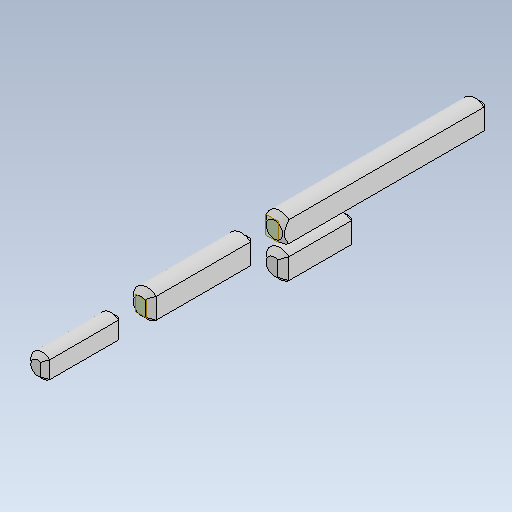
# Autodesk Inventor part: pins
Saved by Autodesk Inventor 2023 (Build 270158030, 158C)
## iProperties
Created: 2024-12-20
Part Number: pins
Material: Generic
Document SubType Name: Modeling
Designer: Imogen Heard
Density: 1 g/cm^3
Appearance: Default
Author: Imogen Heard
Autodesk Inventor part; units mm, degrees
ref_plane "YZ Plane" through (0, 0, 0) normal (1, 0, 0) x (0, 1, 0)
ref_plane "XZ Plane" through (0, 0, 0) normal (0, 1, 0) x (-1, 0, 0)
ref_plane "XY Plane" through (0, 0, 0) normal (0, 0, 1) x (1, 0, 0)
sketch "Sketch1" plane through (0, 0, 0) normal (0, 0, 1) x (1, 0, 0)
  circle A0 centre (-1.65, -26) radius 2.5
  line L0 (-1.65, -28.5) -> (0, -28.5)
  line L1 (0, -28.5) -> (0, -23.5)
  line L2 (0, -23.5) -> (-1.65, -23.5)
  line L3 (-1.65, -23.5) -> (-1.65, -28.5)
  circle A1 centre (-1.65, -38) radius 2.5
  line L4 (-1.65, -40.5) -> (0, -40.5)
  line L5 (0, -40.5) -> (0, -35.5)
  line L6 (0, -35.5) -> (-1.65, -35.5)
  line L7 (-1.65, -35.5) -> (-1.65, -40.5)
  circle A2 centre (-1.65, -44) radius 2.5
  line L8 (-1.65, -46.5) -> (0, -46.5)
  line L9 (0, -46.5) -> (0, -41.5)
  line L10 (0, -41.5) -> (-1.65, -41.5)
  line L11 (-1.65, -41.5) -> (-1.65, -46.5)
  circle A3 centre (-1.65, -32) radius 2.5
  line L12 (-1.65, -34.5) -> (0, -34.5)
  line L13 (0, -34.5) -> (0, -29.5)
  line L14 (0, -29.5) -> (-1.65, -29.5)
  line L15 (-1.65, -29.5) -> (-1.65, -34.5)
  point P0 (0, 0)
  point P1 (0, -27.8782)
  point P2 (0, -24.1218)
  point P3 (0, -33.8782)
  point P4 (0, -30.1218)
  point P5 (0, -39.8782)
  point P6 (0, -36.1218)
  point P7 (0, -45.8782)
  point P8 (0, -42.1218)
  dimension "d0" = 5
  dimension "d1" = 26
  dimension "d2" = 1.65
  dimension "d3" = 5
  dimension "d4" = 1.65
  dimension "d5" = 5
  dimension "d6" = 1.65
  dimension "d7" = 5
  dimension "d8" = 1.65
  dimension "d9" = 6
  dimension "d10" = 6
  dimension "d11" = 6
  constraints: 32 end point, 8 parallel, 8 point on circle, 8 vertical alignment, 4 centre point, 4 horizontal, 4 midpoint, 4 perpendicular
  measures "d0" diameter of A0
  measures "d1" vertical distance of point (0, 0) point (-1.65, -26)
  measures "d2" distance between parallel lines of L1 L3
  measures "d3" diameter of A1
  measures "d4" distance between parallel lines of L5 L7
  measures "d5" diameter of A2
  measures "d6" distance between parallel lines of L9 L11
  measures "d7" diameter of A3
  measures "d8" distance between parallel lines of L13 L15
  measures "d9" distance of A3.centre A0.centre
  measures "d10" distance of point (-1.65, -38) A3.centre
  measures "d11" distance of A1.centre A2.centre
extrude "Extrusion1" add sketch "Sketch1" against normal blind 17 contours L3 A0 | A0 L1 L3
chamfer "Chamfer1" distance 1 angle 45 4 edges at (0, -26, 0) (-4.15, -26, 0) (0, -26, -17) (-4.15, -26, -17)
ref_plane "Work Plane1" through (0, 0, -23) normal (0, 0, -1) x (-1, 0, 0)
sketch "Sketch2" plane through (0, 0, -23) normal (0, 0, -1) x (-1, 0, 0)
  circle A0 centre (1.98, -26) radius 3
  line L0 (1.98, -23) -> (0, -23)
  line L1 (0, -23) -> (0, -29)
  line L2 (0, -29) -> (1.98, -29)
  line L3 (1.98, -29) -> (1.98, -23)
  line L4 (1, -27.3519) -> (1, -24.6481) projected
  circle A1 centre (1.98, -33) radius 3
  line L5 (1.98, -30) -> (0, -30)
  line L6 (0, -30) -> (0, -36)
  line L7 (0, -36) -> (1.98, -36)
  line L8 (1.98, -36) -> (1.98, -30)
  line L9 (1.98, -30) -> (1.98, -36)
  circle A2 centre (1.98, -40) radius 3
  line L10 (1.98, -37) -> (0, -37)
  line L11 (0, -37) -> (0, -43)
  line L12 (0, -43) -> (1.98, -43)
  line L13 (1.98, -43) -> (1.98, -37)
  circle A3 centre (1.98, -47) radius 3
  line L14 (1.98, -44) -> (0, -44)
  line L15 (0, -44) -> (0, -50)
  line L16 (0, -50) -> (1.98, -50)
  line L17 (1.98, -50) -> (1.98, -44)
  line L18 (1.98, -44) -> (1.98, -50)
  line L19 (0, -24.1218) -> (0, -27.8782) projected
  point P0 (0, 0)
  point P1 (1, -26)
  point P2 (0, -26.8782)
  point P3 (1.98, -26)
  point P4 (0, -26.8782)
  point P5 (2.0578, -40)
  point P6 (0, -25.8782)
  point P7 (0, -44.7462)
  point P8 (0, -49.2538)
  point P9 (0, -37.7462)
  point P10 (0, -42.2538)
  point P11 (0, -30.7462)
  point P12 (0, -35.2538)
  point P13 (0, -23.7462)
  point P14 (0, -28.2538)
  dimension "d18" = 6
  dimension "d19" = 1.98
  dimension "d20" = 6
  dimension "d21" = 1.98
  dimension "d22" = 7
  dimension "d23" = 6
  dimension "d24" = 1.98
  dimension "d25" = 6
  dimension "d26" = 1.98
  dimension "d27" = 7
  dimension "d28" = 7
  constraints: 36 end point, 11 vertical alignment, 8 parallel, 8 point on circle, 7 midpoint, 6 coincident, 4 centre point, 4 horizontal, 4 perpendicular, 2 horizontal alignment, 2 vertical
  measures "d18" diameter of A0
  measures "d19" distance between parallel lines of L1 L3
  measures "d20" diameter of A1
  measures "d21" distance between parallel lines of L6 L8
  measures "d22" distance of point (1.98, -33) point (1.98, -26)
  measures "d23" diameter of A2
  measures "d24" distance between parallel lines of L11 L13
  measures "d25" diameter of A3
  measures "d26" distance between parallel lines of L15 L17
  measures "d27" distance of point (1.98, -47) point (1.98, -40)
  measures "d28" vertical distance of point (2.058, -40) A1.centre
extrude "Extrusion2" add sketch "Sketch2" along normal blind 23 separate body contours A0 L3 | L3 A0 L1
chamfer "Chamfer2" distance 1.2 angle 45 4 edges at (-4.98, -26, -23) (0, -26, -23) (-4.98, -26, -46) (0, -26, -46)
ref_plane "Work Plane2" through (0, 0, -52) normal (0, 0, -1) x (-1, 0, 0)
sketch "Sketch3" plane through (0, 0, -52) normal (0, 0, -1) x (-1, 0, 0)
  arc A0 (0, -28.2538) -> (0, -23.7462) centre (1.98, -26) ccw projected
  arc A1 (1.2, -27.6222) -> (1.2, -24.3778) centre (1.98, -26) ccw projected
  line L0 (0, -23.7462) -> (0, -28.2538) projected
  line L1 (1.2, -27.6222) -> (1.2, -24.3778) projected
  arc A2 (0, -35.2538) -> (0, -30.7462) centre (1.98, -33) ccw projected
  arc A3 (1.2, -34.6222) -> (1.2, -31.3778) centre (1.98, -33) ccw projected
  line L2 (1.2, -34.6222) -> (1.2, -31.3778) projected
  arc A4 (1.2, -34.6222) -> (1.2, -31.3778) centre (1.98, -33) ccw projected
  line L3 (1.2, -34.6222) -> (1.2, -31.3778) projected
  line L4 (0, -30.7462) -> (0, -35.2538) projected
  point P0 (0, 0)
  constraints: 6 other
extrude "Extrusion3" add sketch "Sketch3" along normal blind 45 separate body contours L0 A0 | L1 A1
sketch "Sketch4" plane through (0, 0, -52) normal (0, 0, 1) x (1, 0, 0)
  line L0 (0, -35.2538) -> (0, -30.7462) projected
  line L1 (-1.2, -34.6222) -> (-1.2, -31.3778) projected
  arc A0 (-1.2, -31.3778) -> (-1.2, -34.6222) centre (-1.98, -33) ccw projected
  arc A1 (0, -30.7462) -> (0, -35.2538) centre (-1.98, -33) ccw projected
  arc A2 (-1.2, -31.3778) -> (-1.2, -34.6222) centre (-1.98, -33) ccw projected
  line L2 (-1.2, -34.6222) -> (-1.2, -31.3778) projected
  line L3 (0, -30.7462) -> (0, -35.2538) projected
  arc A3 (0, -37.7462) -> (0, -42.2538) centre (-1.98, -40) ccw projected
  arc A4 (-1.2, -38.3778) -> (-1.2, -41.6222) centre (-1.98, -40) ccw projected
  line L4 (-1.2, -41.6222) -> (-1.2, -38.3778) projected
  arc A5 (-1.2, -38.3778) -> (-1.2, -41.6222) centre (-1.98, -40) ccw projected
  line L5 (-1.2, -41.6222) -> (-1.2, -38.3778) projected
  line L6 (0, -37.7462) -> (0, -42.2538) projected
  point P0 (0, 0)
  point P1 (0, -42.2538)
  point P2 (0, -37.7462)
  constraints: 8 other
extrude "Extrusion4" add sketch "Sketch4" against normal blind 16 separate body contours A1 L0 | A0 L1
chamfer "Chamfer3" distance 1.2 angle 45 7 edges at (-4.98, -26, -97) (0, -26, -97) (-4.98, -26, -52) (-4.98, -33, -68) (0, -33, -68) (-4.98, -33, -52) (0, -33, -52)
equation "\"d2\" = 0.33 * d0"
equation "\"d4\" = 0.33 * d3"
equation "\"d6\" = 0.33 * d5"
equation "\"d8\" = 0.33 * d7"
equation "\"d19\" = 0.33 * d18"
equation "\"d21\" = 0.33 * d20"
equation "\"d24\" = 0.33 * d23"
equation "\"d26\" = 0.33 * d25"
